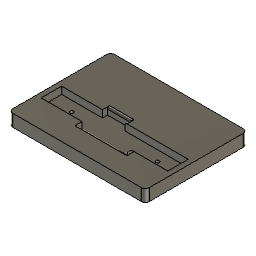
co2_base (Autodesk Fusion 360 design; units mm, degrees)
part number: 2026-03-02-18-48-23-842
Autodesk Fusion 360 part; units mm, degrees
sketch "Sketch1" plane through (0, 0, 0) normal (0, 0, 1) x (1, 0, 0)
  line L0 (0, 0) -> (67, 0)
  line L1 (67, 0) -> (67, 50)
  line L2 (67, 50) -> (0, 50)
  line L3 (0, 50) -> (0, 0)
  dimension "d1" = 67
  dimension "d2" = 50
  constraint horizontal L0
  constraint vertical L1
  constraint horizontal L2
  constraint vertical L3
  constraint coincident L0.start L3.end
  measures "d1" distance of L0.start L0.end
  measures "d2" distance of L0.start L2.end
extrude "Extrude1" add sketch "Sketch1" along normal blind 6
sketch "Sketch2" plane through (0, 0, 6) normal (0, 0, 1) x (-1, 0, 0)
  line L0 (0, -50) -> (0, 0)
  line L1 (0, 0) -> (-67, 0)
  line L2 (-67, 0) -> (-67, -50)
  line L3 (-67, -50) -> (0, -50)
  line L4 (-2.5, -13.5) -> (-64.5, -13.5)
  line L5 (-64.5, -13.5) -> (-64.5, -23.5)
  line L6 (-64.5, -23.5) -> (-2.5, -23.5)
  line L7 (-2.5, -23.5) -> (-2.5, -13.5)
  dimension "d5" = 62
  dimension "d6" = 10
  dimension "d7" = 2.5
  dimension "d8" = 26.5
  constraint horizontal L4
  constraint vertical L5
  constraint horizontal L6
  constraint vertical L7
  measures "d5" distance of L4.start L4.end
  measures "d6" distance of L4.start L6.end
  measures "d7" distance of L0 L7
  measures "d8" distance of L3 L6
extrude "Extrude2" cut sketch "Sketch2" against normal blind 3.5 contours L4 L5 L6 L7
sketch "Sketch3" plane through (0, 0, 6) normal (0, 0, 1) x (-1, 0, 0)
  line L0 (-64.5, -13.5) -> (-2.5, -13.5)
  line L1 (-2.5, -13.5) -> (-2.5, -23.5)
  line L2 (-2.5, -23.5) -> (-64.5, -23.5)
  line L3 (-64.5, -23.5) -> (-64.5, -13.5)
  line L4 (0, -50) -> (0, 0)
  line L5 (0, 0) -> (-67, 0)
  line L6 (-67, 0) -> (-67, -50)
  line L7 (-67, -50) -> (0, -50)
  line L8 (-20, -30) -> (-31, -30)
  line L9 (-31, -30) -> (-31, -7)
  line L10 (-31, -7) -> (-20, -7)
  line L11 (-20, -7) -> (-20, -30)
  arc A0 (-41.0737, -13.5) -> (-31, -7) centre (-43.153, 0.7786) ccw
  line L12 (-41.0737, -13.5) -> (-31, -13.5)
  dimension "d11" = 11
  dimension "d12" = 23
  dimension "d13" = 20
  dimension "d14" = 20
  constraint horizontal L8
  constraint vertical L9
  constraint horizontal L10
  constraint vertical L11
  constraint coincident L0 A0.start
  constraint coincident L0 L12.end
  constraint coincident L9 L12.end
  measures "d11" distance of L8.start L8.end
  measures "d12" distance of L8.start L10.end
  measures "d13" distance of L7 L8
  measures "d14" distance of L4 L11
extrude "Extrude3" cut sketch "Sketch3" against normal blind 3.5 contours L0 L9 L10 L11 | L2 L8 L9 L11
move_face "MoveFace1" by (2.5, 0, 0) 6 faces at (20, 9.1667, 4.8333) (31, 11.3333, 3.6667) (20, 25.6667, 4.8333) (31, 27.8333, 4.8333) (23.6667, 30, 4.8333) (27.3333, 7, 4.8333)
move_face "MoveFace2" by (0, 6.5, 0) 3 faces at (29.8333, 7, 4.8333) (33.5, 11.3333, 4.8333) (22.5, 11.3333, 3.6667)
move_face "MoveFace3" by (0, -4, 0) 3 faces at (33.5, 27.8333, 4.8333) (26.1667, 30, 4.8333) (22.5, 25.6667, 4.8333)
sketch "Sketch4" plane through (0, 0, 6) normal (0, 0, 1) x (-1, 0, 0)
  line L0 (-64.5, -13.5) -> (-2.5, -13.5)
  line L1 (-2.5, -13.5) -> (-2.5, -23.5)
  line L2 (-2.5, -23.5) -> (-22.5, -23.5)
  line L3 (-22.5, -23.5) -> (-22.5, -26)
  line L4 (-22.5, -26) -> (-33.5, -26)
  line L5 (-33.5, -26) -> (-33.5, -23.5)
  line L6 (-33.5, -23.5) -> (-64.5, -23.5)
  line L7 (-64.5, -23.5) -> (-64.5, -13.5)
  line L8 (0, -50) -> (0, 0)
  line L9 (0, 0) -> (-67, 0)
  line L10 (-67, 0) -> (-67, -50)
  line L11 (-67, -50) -> (0, -50)
  line L12 (-22.5, -13.5) -> (-44.5, -13.5)
  line L13 (-44.5, -13.5) -> (-44.5, -11)
  line L14 (-44.5, -11) -> (-22.5, -11)
  line L15 (-22.5, -11) -> (-22.5, -13.5)
  dimension "d17" = 22
  dimension "d18" = 2.5
  dimension "d19" = 22.5
  constraint horizontal L12
  constraint vertical L13
  constraint horizontal L14
  constraint vertical L15
  constraint coincident L0 L12.start
  measures "d17" distance of L12.start L12.end
  measures "d18" distance of L12.start L14.end
  measures "d19" distance of L8 L15
extrude "Extrude4" cut sketch "Sketch4" against normal blind 3.5 contours L0 L12 L13 L14 L15
fillet "Fillet1" radius 1 1 edges at (22.5, 24.75, 6)
fillet "Fillet2" radius 1 1 edges at (27.5, 26, 6)
fillet "Fillet3" radius 1 1 edges at (33.5, 25.25, 6)
fillet "Fillet4" radius 1 1 edges at (33.5, 11, 6)
fillet "Fillet5" radius 3.5 1 edges at (44.5, 11.75, 6)
fillet "Fillet6" radius 2 2 edges at (46.716, 10.6545, 5.7555) (44.7733, 11, 3.8559)
fillet "Fillet9" radius 1 1 edges at (22.5, 11.75, 6)
delete_face "DeleteFace1" 1 faces at (21.7822, 11.3541, 5.9594)
delete_face "DeleteFace2" 1 faces at (21.7822, 25.6459, 5.9594)
fillet "Fillet10" radius 2 1 edges at (67, 0, 3)
fillet "Fillet11" radius 2 1 edges at (0, 0, 3)
fillet "Fillet12" radius 2 1 edges at (67, 50, 3)
fillet "Fillet13" radius 2 1 edges at (0, 50, 3)
hole "Hole1" at (12.5, 18.5, 0) direction (0, 0, 1) diameter 1.8 end through all countersink diameter 3.8 countersink angle 90
hole "Hole2" at (54.5, 18.5, 0) direction (0, 0, 1) diameter 1.8 end through all countersink diameter 3.8 countersink angle 90
